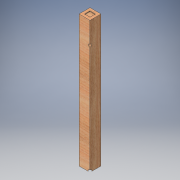
# Autodesk Inventor part: LegOutlet
Saved by Autodesk Inventor 2016 (Build 200138000, 138)
## iProperties
Created: 2016-02-09
Part Number: LegOutlet
Material: Wood (Birch)
Document SubType Name: Modeling
Designer: ron
Density: 0.55 g/cm^3
Appearance: Birch - Natural Polished
Mass: 823.456 g
Surface Area: 1517.67 cm^2
Volume: 1497.19 cm^3
Author: ron
Autodesk Inventor part; units mm, degrees
ref_plane "YZ Plane" through (0, 0, 0) normal (1, 0, 0) x (0, 1, 0)
ref_plane "XZ Plane" through (0, 0, 0) normal (0, 1, 0) x (-1, 0, 0)
ref_plane "XY Plane" through (0, 0, 0) normal (0, 0, 1) x (1, 0, 0)
sketch "Sketch1" plane through (0, 0, 0) normal (1, 0, 0) x (0, 1, 0)
  line L0 (0, 0) -> (609.6, 0)
  line L1 (609.6, 0) -> (609.6, -50.8)
  line L2 (609.6, -50.8) -> (0, -50.8)
  line L3 (0, -50.8) -> (0, 0)
  dimension "d0" = 609.6
  dimension "d1" = 50.8
  constraints: 8 end point, 2 parallel, 1 horizontal, 1 perpendicular
  measures "d0" distance of L1.end L2.end
  measures "d1" distance of L0.end L1.end
extrude "Extrusion1" add sketch "Sketch1" along normal blind 50.8
ref_plane "Work Plane2" through (50.8, 0, 0) normal (0.7071068, 0, 0.7071068) x (0, -1, 0)
sketch "Sketch4" plane through (50.8, 0, 0) normal (0.7071068, 0, 0.7071068) x (0, -1, 0)
  line L0 (-609.6, 0) -> (-508, 0)
  line L1 (0, 0) -> (-3.175, 0)
  point P0 (0, -35.921)
  dimension "d8" = 101.6
  dimension "d16" = 3.175
  constraints: 4 end point
  measures "d8" distance of L0.start L0.end
  measures "d16" distance of L1.start L1.end
hole "Hole1" at (50.8, 508, 0) direction (-0.7071068, 0, -0.7071068) diameter 11.1125 depth 35.9156
sketch "Sketch6" plane through (50.8, 0, 0) normal (0.7071068, 0, 0.7071068) x (0, -1, 0)
  line L0 (0, -35.921) -> (0, 0) projected
  line L1 (0, 0) -> (-3.175, 0)
  line L2 (-609.6, 0) -> (0, 0) projected
  dimension "d17" = 3.175
  constraints: 2 end point, 1 point on line
  measures "d17" distance of L0.end L1.end
hole "Hole2" at (50.8, 3.175, 0) direction (-0.7071068, 0, -0.7071068) diameter 12.7 depth 42.2656
sketch "Sketch10" plane through (0, 0, -50.8) normal (0, -1, 0) x (1, 0, 0)
  line L0 (0, 0) -> (25.3962, 25.3962)
  line L1 (0, 0) -> (50.8, 0) projected
  point P0 (0, 50.8)
  point P1 (50.8, 50.8)
  dimension "d34" = 35.9156
  dimension "d35" = 45
  constraints: 2 end point
  measures "d34" distance of L0.start L0.end
  measures "d35" angle of L1 L0
hole "Hole4" at (25.3962, 0, -25.4038) direction (0, 1, 0) diameter 12.7 depth 538.9626
sketch "Sketch11" plane through (0, 609.6, 0) normal (0, 1, 0) x (1, 0, 0)
  line L0 (12.7, 38.1) -> (38.1, 38.1)
  line L1 (38.1, 38.1) -> (38.1, 12.7)
  line L2 (38.1, 12.7) -> (12.7, 12.7)
  line L3 (12.7, 12.7) -> (12.7, 38.1)
  line L4 (0, 50.8) -> (0, 0) projected
  line L5 (0, 50.8) -> (50.8, 50.8) projected
  dimension "d43" = 25.4
  dimension "d44" = 25.4
  dimension "d45" = 12.7
  dimension "d46" = 12.7
  constraints: 8 end point, 2 parallel, 1 horizontal, 1 perpendicular
  measures "d43" distance of L1.end L2.end
  measures "d44" distance of L0.end L1.end
  measures "d45" distance between parallel lines of L4 L3
  measures "d46" distance between parallel lines of L5 L0
extrude "Extrusion2" cut sketch "Sketch11" against normal blind 3.175
body "Solid1"
